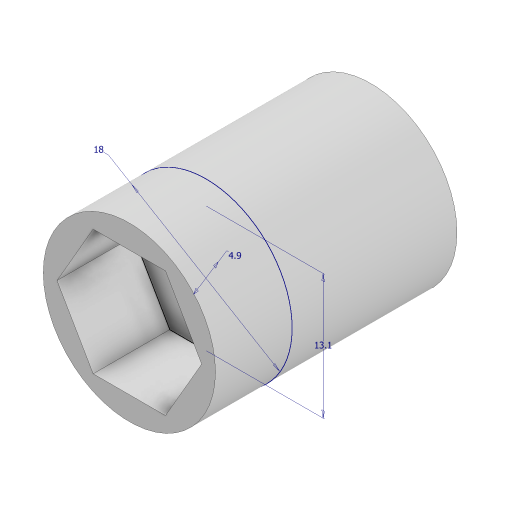
# Autodesk Inventor part: End Shaft Spacers
Saved by Autodesk Inventor 2023 (Build 270158000, 158)
## iProperties
Created: 2023-01-19
Part Number: End Shaft Spacers
Material: Generic
Document SubType Name: Modeling
Designer: david
Density: 1 g/cm^3
Appearance: Default
Author: david
Autodesk Inventor part; units mm, degrees
ref_plane "YZ Plane" through (0, 0, 0) normal (1, 0, 0) x (0, 1, 0)
ref_plane "XZ Plane" through (0, 0, 0) normal (0, 1, 0) x (-1, 0, 0)
ref_plane "XY Plane" through (0, 0, 0) normal (0, 0, 1) x (1, 0, 0)
sketch "Sketch1" plane through (0, 0, 0) normal (0, 0, 1) x (1, 0, 0)
  line L0 (-7.5633, 0) -> (-3.7816, 6.55)
  line L1 (-3.7816, 6.55) -> (3.7816, 6.55)
  line L2 (3.7816, 6.55) -> (7.5633, 0)
  line L3 (7.5633, 0) -> (3.7816, -6.55)
  line L4 (3.7816, -6.55) -> (-3.7816, -6.55)
  line L5 (-3.7816, -6.55) -> (-7.5633, 0)
  circle A0 centre (0, 0) radius 9
  circle A1 centre (0, 0) radius 2.45
  point P0 (0, -6.55)
  point P1 (0, 6.55)
  dimension "d0" = 13.1
  dimension "d1" = 18
  dimension "d2" = 4.9
  constraints: 12 end point, 3 coincident, 2 centre point, 2 midpoint, 13 other
  measures "d0" distance of point (0, -6.55) point (0, 6.55)
  measures "d1" diameter of A0
  measures "d2" diameter of A1
extrude "Extrusion1" add sketch "Sketch1" along normal blind 8 contours A0
extrude "Extrusion2" add sketch "Sketch1" against normal blind 17.25 contours L0 L1 L2 L3 L4 L5 | A0
sketch "Sketch2" plane through (0, 0, -17.25) normal (0, 0, -1) x (-1, 0, 0)
  circle A0 centre (0, 0) radius 5
  dimension "d7" = 10
  constraints: 1 centre point, 1 coincident
  measures "d7" diameter of A0
extrude "Extrusion3" cut sketch "Sketch2" against normal blind 12.75
body "Solid1"
